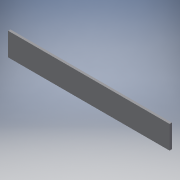
# Autodesk Inventor part: basePlate
Saved by Autodesk Inventor 2019 (Build 230136000, 136)
## iProperties
Created: 2021-11-19
Part Number: basePlate
Material: Generic
Document SubType Name: Modeling
Designer: Pokick
Density: 1 g/cm^3
Appearance: Default
Author: Pokick
Autodesk Inventor part; units mm, degrees
ref_plane "YZ Plane" through (0, 0, 0) normal (1, 0, 0) x (0, 1, 0)
ref_plane "XZ Plane" through (0, 0, 0) normal (0, 1, 0) x (-1, 0, 0)
ref_plane "XY Plane" through (0, 0, 0) normal (0, 0, 1) x (1, 0, 0)
sketch "Sketch1" plane through (0, 0, 0) normal (0, 0, 1) x (1, 0, 0)
  line L0 (0, 0) -> (500, 0) construction
  line L1 (500, 0) -> (500, 10) construction
  line L2 (500, 10) -> (0, 10) construction
  line L3 (0, 10) -> (0, 0) construction
  line L4 (250, 0) -> (250, 10) construction
  line L5 (500, -45) -> (0, -45)
  line L6 (0, -45) -> (0, 55)
  line L7 (0, 55) -> (500, 55)
  line L8 (500, 55) -> (500, -45)
  line L9 (500, -45) -> (0, 55) construction
  line L10 (0, -45) -> (500, 55) construction
  line L11 (0, 55) -> (-200, 55)
  line L12 (-200, 55) -> (-200, -45)
  line L13 (-200, -45) -> (0, -45)
  line L14 (0, -45) -> (0, 55)
  point P0 (250, 5)
  dimension "d0" = 500
  dimension "d1" = 10
  dimension "d2" = 500
  dimension "d3" = 100
  dimension "d4" = 200
  dimension "d5" = 100
  constraints: 30 end point, 6 parallel, 5 midpoint, 3 horizontal, 3 perpendicular
  measures "d0" distance of L2.end L1.end
  measures "d1" distance of L1.end L0.end
  measures "d2" distance of L6.end L7.end
  measures "d3" distance of L5.end L6.end
  measures "d4" distance of L13.end L12.end
  measures "d5" distance of L12.end L11.end
extrude "Extrusion1" add sketch "Sketch1" along normal blind 10
body "Solid1"
